# Autodesk Inventor part: 4_7UF
Saved by Autodesk Inventor 2016 SP1 (Build 200210100, 210)
## iProperties
Created: 2015-11-19
Part Number: 4_7UF
Material: Generic
Document SubType Name: Modeling
Designer: PhillipD
Density: 1 g/cm^3
Appearance: 0603-CAP, 4_7UF
Author: PhillipD
Autodesk Inventor part; units mm, degrees
ref_plane "YZ Plane" through (0, 0, 0) normal (1, 0, 0) x (0, 1, 0)
ref_plane "XZ Plane" through (0, 0, 0) normal (0, 1, 0) x (-1, 0, 0)
ref_plane "XY Plane" through (0, 0, 0) normal (0, 0, 1) x (1, 0, 0)
sketch "0603-CAP, 4_7UF_10" plane through (0, 0, 0) normal (0, 0, 1) x (1, 0, 0)
  line L0 (-1.4984, 1.0084) -> (1.4984, 1.0084)
  line L1 (1.4984, 1.0084) -> (1.4984, -0.983)
  line L2 (1.4984, -0.983) -> (-1.4984, -0.983)
  line L3 (-1.4984, -0.983) -> (-1.4984, 1.0084)
  constraints: 8 end point
extrude "Extrusion1" add sketch "0603-CAP, 4_7UF_10" along normal blind 1
body "Solid1"
